Autodesk Fusion 360 part; units mm, degrees
(part 5 of 5)
  arc A59 (-253.4198, 76.6618) -> (-253.4094, 76.4118) centre (-250.4198, 76.6618) ccw
  line L124 (-253.4198, 76.6618) -> (-253.4198, 77.4318)
  arc A60 (-253.4094, 77.6818) -> (-253.4198, 77.4318) centre (-250.4198, 77.4318) ccw
  arc A61 (-253.4198, 77.9318) -> (-253.4094, 77.6818) centre (-250.4198, 77.9318) ccw
  line L125 (-253.4198, 77.9318) -> (-253.4198, 78.7018)
  arc A62 (-253.4094, 78.9518) -> (-253.4198, 78.7018) centre (-250.4198, 78.7018) ccw
  arc A63 (-253.4198, 79.2018) -> (-253.4094, 78.9518) centre (-250.4198, 79.2018) ccw
  line L126 (-253.4198, 79.2018) -> (-253.4198, 79.9718)
  arc A64 (-253.4094, 80.2218) -> (-253.4198, 79.9718) centre (-250.4198, 79.9718) ccw
  arc A65 (-253.4198, 80.4718) -> (-253.4094, 80.2218) centre (-250.4198, 80.4718) ccw
  line L127 (-253.4198, 80.4718) -> (-253.4198, 85.5518)
  arc A66 (-252.4198, 86.5518) -> (-253.4198, 85.5518) centre (-252.4198, 85.5518) ccw
  line L128 (-252.4198, 86.5518) -> (-249.2148, 86.5518)
  arc A67 (-248.9648, 86.5414) -> (-249.2148, 86.5518) centre (-249.2148, 83.5518) ccw
  arc A68 (-248.7148, 86.5518) -> (-248.9648, 86.5414) centre (-248.7148, 83.5518) ccw
  line L129 (-333.4198, 66.966) -> (-333.4198, 73.5518)
  line L130 (-333.4198, 73.5518) -> (-326.834, 73.5518)
  line L131 (-326.834, 73.5518) -> (-333.4198, 66.966)
  line L132 (-323.4198, 72.1376) -> (-316.834, 65.5518)
  line L133 (-316.834, 65.5518) -> (-323.4198, 65.5518)
  line L134 (-323.4198, 65.5518) -> (-323.4198, 72.1376)
  line L135 (-305.4198, 72.1376) -> (-305.4198, 65.5518)
  line L136 (-305.4198, 65.5518) -> (-312.0056, 65.5518)
  line L137 (-312.0056, 65.5518) -> (-305.4198, 72.1376)
  line L138 (-303.4198, 76.966) -> (-303.4198, 83.5518)
  line L139 (-303.4198, 83.5518) -> (-296.834, 83.5518)
  line L140 (-296.834, 83.5518) -> (-303.4198, 76.966)
  line L141 (-285.4198, 65.5518) -> (-292.0056, 65.5518)
  line L142 (-292.0056, 65.5518) -> (-285.4198, 72.1376)
  line L143 (-285.4198, 72.1376) -> (-285.4198, 65.5518)
  line L144 (-283.4198, 83.5518) -> (-276.834, 83.5518)
  line L145 (-276.834, 83.5518) -> (-283.4198, 76.966)
  line L146 (-283.4198, 76.966) -> (-283.4198, 83.5518)
  line L147 (-265.4198, 65.5518) -> (-272.0056, 65.5518)
  line L148 (-272.0056, 65.5518) -> (-265.4198, 72.1376)
  line L149 (-265.4198, 72.1376) -> (-265.4198, 65.5518)
  line L150 (-263.4198, 76.966) -> (-263.4198, 83.5518)
  line L151 (-263.4198, 83.5518) -> (-256.834, 83.5518)
  line L152 (-256.834, 83.5518) -> (-263.4198, 76.966)
  line L153 (-262.0056, 73.5518) -> (-255.4198, 73.5518)
  line L154 (-255.4198, 73.5518) -> (-255.4198, 66.966)
  line L155 (-255.4198, 66.966) -> (-262.0056, 73.5518)
  line L156 (-272.0056, 83.5518) -> (-265.4198, 83.5518)
  line L157 (-265.4198, 83.5518) -> (-265.4198, 76.966)
  line L158 (-265.4198, 76.966) -> (-272.0056, 83.5518)
  line L159 (-282.0056, 73.5518) -> (-275.4198, 73.5518)
  line L160 (-275.4198, 73.5518) -> (-275.4198, 66.966)
  line L161 (-275.4198, 66.966) -> (-282.0056, 73.5518)
  line L162 (-285.4198, 76.966) -> (-292.0056, 83.5518)
  line L163 (-292.0056, 83.5518) -> (-285.4198, 83.5518)
  line L164 (-285.4198, 83.5518) -> (-285.4198, 76.966)
  line L165 (-302.0056, 73.5518) -> (-295.4198, 73.5518)
  line L166 (-295.4198, 73.5518) -> (-295.4198, 66.966)
  line L167 (-295.4198, 66.966) -> (-302.0056, 73.5518)
  line L168 (-305.4198, 76.966) -> (-312.0056, 83.5518)
  line L169 (-312.0056, 83.5518) -> (-305.4198, 83.5518)
  line L170 (-305.4198, 83.5518) -> (-305.4198, 76.966)
  line L171 (-315.4198, 66.966) -> (-322.0056, 73.5518)
  line L172 (-322.0056, 73.5518) -> (-315.4198, 73.5518)
  line L173 (-315.4198, 73.5518) -> (-315.4198, 66.966)
  line L174 (-325.4198, 65.5518) -> (-332.0056, 65.5518)
  line L175 (-332.0056, 65.5518) -> (-325.4198, 72.1376)
  line L176 (-325.4198, 72.1376) -> (-325.4198, 65.5518)
  line L177 (-332.0056, 83.5518) -> (-325.4198, 83.5518)
  line L178 (-325.4198, 83.5518) -> (-325.4198, 76.966)
  line L179 (-325.4198, 76.966) -> (-332.0056, 83.5518)
  line L180 (-323.4198, 76.966) -> (-323.4198, 83.5518)
  line L181 (-323.4198, 83.5518) -> (-316.834, 83.5518)
  line L182 (-316.834, 83.5518) -> (-323.4198, 76.966)
  line L183 (-313.4198, 66.966) -> (-313.4198, 73.5518)
  line L184 (-313.4198, 73.5518) -> (-306.834, 73.5518)
  line L185 (-306.834, 73.5518) -> (-313.4198, 66.966)
  line L186 (-303.4198, 72.1376) -> (-296.834, 65.5518)
  line L187 (-296.834, 65.5518) -> (-303.4198, 65.5518)
  line L188 (-303.4198, 65.5518) -> (-303.4198, 72.1376)
  line L189 (-293.4198, 66.966) -> (-293.4198, 73.5518)
  line L190 (-293.4198, 73.5518) -> (-286.834, 73.5518)
  line L191 (-286.834, 73.5518) -> (-293.4198, 66.966)
  line L192 (-282.0056, 75.5518) -> (-275.4198, 82.1376)
  line L193 (-275.4198, 82.1376) -> (-275.4198, 75.5518)
  line L194 (-275.4198, 75.5518) -> (-282.0056, 75.5518)
  line L195 (-273.4198, 66.966) -> (-273.4198, 73.5518)
  line L196 (-273.4198, 73.5518) -> (-266.834, 73.5518)
  line L197 (-266.834, 73.5518) -> (-273.4198, 66.966)
  line L198 (-262.0056, 75.5518) -> (-255.4198, 82.1376)
  line L199 (-255.4198, 82.1376) -> (-255.4198, 75.5518)
  line L200 (-255.4198, 75.5518) -> (-262.0056, 75.5518)
  line L201 (-263.4198, 65.5518) -> (-263.4198, 72.1376)
  line L202 (-263.4198, 72.1376) -> (-256.834, 65.5518)
  line L203 (-256.834, 65.5518) -> (-263.4198, 65.5518)
  line L204 (-273.4198, 82.1376) -> (-266.834, 75.5518)
  line L205 (-266.834, 75.5518) -> (-273.4198, 75.5518)
  line L206 (-273.4198, 75.5518) -> (-273.4198, 82.1376)
  line L207 (-283.4198, 65.5518) -> (-283.4198, 72.1376)
  line L208 (-283.4198, 72.1376) -> (-276.834, 65.5518)
  line L209 (-276.834, 65.5518) -> (-283.4198, 65.5518)
  line L210 (-293.4198, 82.1376) -> (-286.834, 75.5518)
  line L211 (-286.834, 75.5518) -> (-293.4198, 75.5518)
  line L212 (-293.4198, 75.5518) -> (-293.4198, 82.1376)
  line L213 (-302.0056, 75.5518) -> (-295.4198, 82.1376)
  line L214 (-295.4198, 82.1376) -> (-295.4198, 75.5518)
  line L215 (-295.4198, 75.5518) -> (-302.0056, 75.5518)
  line L216 (-313.4198, 75.5518) -> (-313.4198, 82.1376)
  line L217 (-313.4198, 82.1376) -> (-306.834, 75.5518)
  line L218 (-306.834, 75.5518) -> (-313.4198, 75.5518)
  line L219 (-322.0056, 75.5518) -> (-315.4198, 82.1376)
  line L220 (-315.4198, 82.1376) -> (-315.4198, 75.5518)
  line L221 (-315.4198, 75.5518) -> (-322.0056, 75.5518)
  line L222 (-333.4198, 82.1376) -> (-326.834, 75.5518)
  line L223 (-326.834, 75.5518) -> (-333.4198, 75.5518)
  line L224 (-333.4198, 75.5518) -> (-333.4198, 82.1376)
  line L225 (-278.3217, 111.8636) -> (-280.8652, 114.4071)
  line L226 (-278.3217, 106.2068) -> (-286.4809, 114.3659)
  line L227 (-278.3217, 100.5499) -> (-292.089, 114.3172)
  line L228 (-278.3217, 94.893) -> (-297.693, 114.2643)
  line L229 (-278.3217, 89.2362) -> (-303.3266, 114.2411)
  line L230 (-283.9362, 89.1938) -> (-308.9411, 114.1987)
  line L231 (-289.5507, 89.1515) -> (-314.5556, 114.1564)
  line L232 (-333.4198, 103.3404) -> (-322.6241, 114.1362)
  line L233 (-333.4198, 108.9972) -> (-328.2809, 114.1362)
  line L234 (-325.0115, 89.1213) -> (-311.4909, 102.6419)
  line L235 (-330.6683, 89.1213) -> (-314.3193, 105.4703)
  line L236 (-333.4208, 92.0257) -> (-317.1477, 108.2988)
  line L237 (-333.4198, 97.6835) -> (-319.9762, 111.1272)
  line L238 (-319.3546, 89.1213) -> (-308.6625, 99.8135)
  line L239 (-313.6978, 77.8076) -> (-307.9536, 83.5518)
  line L240 (-302.3841, 89.1213) -> (-300.1772, 91.3282)
  line L241 (-316.5262, 80.636) -> (-315.4198, 81.7424)
  line L242 (-308.0409, 89.1213) -> (-303.0056, 94.1566)
  line L243 (-319.3546, 83.4645) -> (-319.2673, 83.5518)
  line L244 (-313.6978, 89.1213) -> (-305.834, 96.985)
  line L245 (-277.6146, 112.5707) -> (-280.1581, 115.1143)
  line L246 (-279.0288, 111.1565) -> (-281.5724, 113.7)
  line L247 (-277.6146, 106.9139) -> (-285.7738, 115.073)
  line L248 (-279.0288, 105.4996) -> (-287.188, 113.6588)
  line L249 (-277.6146, 101.257) -> (-291.3819, 115.0243)
  line L250 (-279.0288, 99.8428) -> (-292.7961, 113.6101)
  line L251 (-277.6146, 95.6002) -> (-296.9859, 114.9714)
  line L252 (-279.0288, 94.1859) -> (-298.4001, 113.5572)
  line L253 (-277.6146, 89.9433) -> (-302.6195, 114.9482)
  line L254 (-279.0288, 88.5291) -> (-304.0337, 113.534)
  line L255 (-283.2291, 89.9009) -> (-308.234, 114.9058)
  line L256 (-284.6433, 88.4867) -> (-309.6482, 113.4916)
  line L257 (-288.8436, 89.8586) -> (-313.8485, 114.8635)
  line L258 (-290.2578, 88.4444) -> (-315.2627, 113.4493)
  line L259 (-301.677, 88.4142) -> (-299.4701, 90.6211)
  line L260 (-303.0912, 89.8284) -> (-300.8843, 92.0353)
  line L261 (-307.3338, 88.4142) -> (-302.2985, 93.4495)
  line L262 (-308.748, 89.8284) -> (-303.7127, 94.8637)
  line L263 (-312.9907, 88.4142) -> (-305.1269, 96.2779)
  line L264 (-314.4049, 89.8284) -> (-306.5411, 97.6922)
  line L265 (-318.6475, 88.4142) -> (-307.9554, 99.1064)
  line L266 (-320.0617, 89.8284) -> (-309.3696, 100.5206)
  line L267 (-324.3044, 88.4142) -> (-310.7838, 101.9348)
  line L268 (-325.7186, 89.8284) -> (-312.198, 103.349)
  line L269 (-329.9612, 88.4142) -> (-313.6122, 104.7632)
  line L270 (-331.3754, 89.8284) -> (-315.0264, 106.1774)
  line L271 (-332.7137, 91.3186) -> (-316.4406, 107.5916)
  line L272 (-334.1279, 92.7328) -> (-317.8549, 109.0059)
  line L273 (-332.7127, 96.9764) -> (-319.2691, 110.4201)
  line L274 (-334.1269, 98.3906) -> (-320.6833, 111.8343)
  line L275 (-332.7127, 102.6333) -> (-321.917, 113.429)
  line L276 (-334.1269, 104.0475) -> (-323.3312, 114.8433)
  line L277 (-332.7127, 108.2901) -> (-327.5738, 113.429)
  line L278 (-334.1269, 109.7043) -> (-328.988, 114.8433)
  circle A69 centre (-278.3217, 111.8636) radius 1
  circle A70 centre (-280.8652, 114.4071) radius 1
  circle A71 centre (-286.4809, 114.3659) radius 1
  circle A72 centre (-292.089, 114.3172) radius 1
  circle A73 centre (-297.693, 114.2643) radius 1
  circle A74 centre (-303.3266, 114.2411) radius 1
  circle A75 centre (-308.9411, 114.1987) radius 1
  circle A76 centre (-314.5556, 114.1564) radius 1
  circle A77 centre (-328.2809, 114.1362) radius 1
  circle A78 centre (-322.6241, 114.1362) radius 1
  circle A79 centre (-319.9762, 111.1272) radius 1
  circle A80 centre (-317.1477, 108.2988) radius 1
  circle A81 centre (-314.3193, 105.4703) radius 1
  circle A82 centre (-311.4909, 102.6419) radius 1
  circle A83 centre (-308.6625, 99.8135) radius 1
  circle A84 centre (-305.834, 96.985) radius 1
  circle A85 centre (-303.0056, 94.1566) radius 1
  circle A86 centre (-300.1772, 91.3282) radius 1
  circle A87 centre (-333.4198, 97.6835) radius 1
  circle A88 centre (-333.4198, 103.3404) radius 1
  circle A89 centre (-333.4198, 108.9972) radius 1
  circle A90 centre (-333.4208, 92.0257) radius 1
  circle A91 centre (-330.6683, 89.1213) radius 1
  circle A92 centre (-325.0115, 89.1213) radius 1
  circle A93 centre (-319.3546, 89.1213) radius 1
  circle A94 centre (-313.6978, 89.1213) radius 1
  circle A95 centre (-308.0409, 89.1213) radius 1
  circle A96 centre (-302.3841, 89.1213) radius 1
  circle A97 centre (-289.5507, 89.1515) radius 1
  circle A98 centre (-283.9362, 89.1938) radius 1
  circle A99 centre (-278.3217, 89.2362) radius 1
  circle A100 centre (-278.3217, 94.893) radius 1
  circle A101 centre (-278.3217, 100.5499) radius 1
  circle A102 centre (-278.3217, 106.2068) radius 1
  spline S197 degree 3 poles (-269.4518, 103.3713) (-269.4881, 103.3939) (-269.5678, 103.4435) (-269.6619, 103.4471) (-269.713, 103.4491) knots 0 0 0 0 0.012631 0.027679 0.027679 0.027679 0.027679
  spline S198 degree 3 poles (-270.0459, 103.2185) (-270.0428, 103.1922) (-270.0364, 103.1388) (-269.9947, 103.1048) (-269.9736, 103.0875) knots 0 0 0 0 0.007652 0.015492 0.015492 0.015492 0.015492
  spline S199 degree 3 poles (-269.9736, 103.0875) (-269.9445, 103.0745) (-269.8638, 103.0382) (-269.7777, 103.0175) (-269.7226, 103.0043) knots 0 0 0 0 0.009553 0.026493 0.026493 0.026493 0.026493
  spline S200 degree 3 poles (-269.7226, 103.0043) (-269.6457, 102.9851) (-269.5185, 102.9532) (-269.3964, 102.9053) (-269.3481, 102.8863) knots 0 0 0 0 0.023736 0.039299 0.039299 0.039299 0.039299
  spline S201 degree 3 poles (-269.3481, 102.8863) (-269.3157, 102.8686) (-269.2528, 102.8342) (-269.2104, 102.7765) (-269.1898, 102.7485) knots 0 0 0 0 0.010927 0.021211 0.021211 0.021211 0.021211
  spline S202 degree 3 poles (-269.1898, 102.7485) (-269.1741, 102.7183) (-269.1424, 102.6573) (-269.1381, 102.5887) (-269.1359, 102.5541) knots 0 0 0 0 0.010103 0.020373 0.020373 0.020373 0.020373
  spline S203 degree 3 poles (-269.1359, 102.5541) (-269.1377, 102.5225) (-269.1413, 102.46) (-269.1674, 102.403) (-269.1803, 102.3747) knots 0 0 0 0 0.009394 0.018625 0.018625 0.018625 0.018625
  spline S204 degree 3 poles (-269.1803, 102.3747) (-269.1964, 102.3484) (-269.2287, 102.2956) (-269.2769, 102.257) (-269.301, 102.2376) knots 0 0 0 0 0.009191 0.018392 0.018392 0.018392 0.018392
  spline S205 degree 3 poles (-269.301, 102.2376) (-269.3232, 102.2237) (-269.372, 102.1929) (-269.4271, 102.1755) (-269.4572, 102.166) knots 0 0 0 0 0.007816 0.017247 0.017247 0.017247 0.017247
  line L279 (-270.6352, 51.6914) -> (-270.3788, 51.6914)
  spline S206 degree 3 poles (-271.2001, 103.4491) (-271.2429, 103.4465) (-271.3256, 103.4416) (-271.3964, 103.3988) (-271.4306, 103.3781) knots 0 0 0 0 0.012642 0.024448 0.024448 0.024448 0.024448
  spline S207 degree 3 poles (-271.6134, 103.5282) (-271.5534, 103.564) (-271.4259, 103.6399) (-271.2773, 103.6472) (-271.1987, 103.651) knots 0 0 0 0 0.020652 0.043844 0.043844 0.043844 0.043844
  spline S208 degree 3 poles (-270.6967, 102.3386) (-270.7652, 102.2797) (-270.9056, 102.1591) (-271.0905, 102.1442) (-271.1851, 102.1367) knots 0 0 0 0 0.026399 0.05408 0.05408 0.05408 0.05408
  spline S209 degree 3 poles (-271.1851, 102.1367) (-271.2768, 102.1442) (-271.4567, 102.159) (-271.593, 102.2768) (-271.6598, 102.3345) knots 0 0 0 0 0.026858 0.052633 0.052633 0.052633 0.052633
  spline S210 degree 3 poles (-271.6598, 102.3345) (-271.7135, 102.4112) (-271.8298, 102.5776) (-271.839, 102.7813) (-271.844, 102.8911) knots 0 0 0 0 0.027523 0.05971 0.05971 0.05971 0.05971
  spline S211 degree 3 poles (-271.844, 102.8911) (-271.8439, 102.9002) (-271.8437, 102.922) (-271.843, 102.9438) (-271.8426, 102.9566) knots 0 0 0 0 0.002729 0.00655 0.00655 0.00655 0.00655
  line L280 (-271.8426, 102.9566) -> (-270.7621, 102.9566)
  spline S212 degree 3 poles (-270.7621, 102.9566) (-270.7692, 103.0293) (-270.7823, 103.1635) (-270.8611, 103.2724) (-270.8972, 103.3222) knots 0 0 0 0 0.021465 0.039604 0.039604 0.039604 0.039604
  spline S213 degree 3 poles (-272.4886, 103.3904) (-272.5003, 103.3956) (-272.527, 103.4073) (-272.5562, 103.4078) (-272.5725, 103.4081) knots 0 0 0 0 0.003804 0.008651 0.008651 0.008651 0.008651
  spline S214 degree 3 poles (-272.7158, 103.6155) (-272.6831, 103.6219) (-272.6218, 103.6338) (-272.5594, 103.6362) (-272.5302, 103.6373) knots 0 0 0 0 0.009958 0.018706 0.018706 0.018706 0.018706
  spline S215 degree 3 poles (-272.2192, 103.4839) (-272.2105, 103.4484) (-272.1875, 103.3534) (-272.1885, 103.2553) (-272.1892, 103.194) knots 0 0 0 0 0.010927 0.02924 0.02924 0.02924 0.02924
  line L281 (-272.1892, 103.194) -> (-272.1892, 102.3604)
  line L282 (-272.1892, 102.3604) -> (-272.0091, 102.3604)
  line L283 (-272.0091, 102.3604) -> (-272.0091, 102.1694)
  line L284 (-272.0091, 102.1694) -> (-272.1892, 102.1694)
  line L285 (-272.1892, 102.1694) -> (-272.1892, 101.8106)
  line L286 (-272.1892, 101.8106) -> (-272.4334, 101.6633)
  line L287 (-272.4334, 101.6633) -> (-272.4334, 102.1694)
  line L288 (-272.4334, 102.1694) -> (-272.6803, 102.1694)
  line L289 (-272.6803, 102.1694) -> (-272.6803, 102.3604)
  line L290 (-272.6803, 102.3604) -> (-272.4334, 102.3604)
  line L291 (-272.4334, 102.3604) -> (-272.4334, 103.2076)
  spline S216 degree 3 poles (-272.4334, 103.2076) (-272.433, 103.2365) (-272.4324, 103.2821) (-272.4426, 103.3265) (-272.4463, 103.3427) knots 0 0 0 0 0.008635 0.013608 0.013608 0.013608 0.013608
  spline S217 degree 3 poles (-272.4463, 103.3427) (-272.4514, 103.3522) (-272.4616, 103.3715) (-272.4795, 103.384) (-272.4886, 103.3904) knots 0 0 0 0 0.003189 0.00646 0.00646 0.00646 0.00646
  line L292 (-265.9218, 102.7301) -> (-265.9218, 103.6182)
  line L293 (-265.6571, 101.6182) -> (-266.5439, 101.6182)
  spline S218 degree 3 poles (-266.5439, 101.6182) (-266.6229, 101.6188) (-266.7608, 101.6199) (-266.8937, 101.6565) (-266.9504, 101.6721) knots 0 0 0 0 0.023572 0.041164 0.041164 0.041164 0.041164
  spline S219 degree 3 poles (-267.256, 102.1639) (-267.2506, 102.2317) (-267.2401, 102.365) (-267.1584, 102.4707) (-267.1182, 102.5227) knots 0 0 0 0 0.019911 0.039185 0.039185 0.039185 0.039185
  line L294 (-267.0868, 103.6182) -> (-266.8222, 103.2021)
  spline S220 degree 3 poles (-266.8222, 103.2021) (-266.7876, 103.1487) (-266.7268, 103.0548) (-266.66, 102.9652) (-266.6312, 102.9266) knots 0 0 0 0 0.019089 0.033538 0.033538 0.033538 0.033538
  spline S221 degree 3 poles (-266.6312, 102.9266) (-266.6086, 102.8983) (-266.5688, 102.8486) (-266.5185, 102.8097) (-266.4968, 102.7929) knots 0 0 0 0 0.010792 0.019015 0.019015 0.019015 0.019015
  spline S222 degree 3 poles (-266.4968, 102.7929) (-266.4772, 102.7812) (-266.4392, 102.7584) (-266.3967, 102.7458) (-266.3761, 102.7397) knots 0 0 0 0 0.006806 0.01324 0.01324 0.01324 0.01324
  spline S223 degree 3 poles (-266.3761, 102.7397) (-266.3563, 102.7369) (-266.3075, 102.7301) (-266.2581, 102.7301) (-266.2287, 102.7301) knots 0 0 0 0 0.005978 0.01478 0.01478 0.01478 0.01478
  line L295 (-266.2287, 102.7301) -> (-265.9218, 102.7301)
  line L296 (-268.8917, 102.9566) -> (-267.8113, 102.9566)
  spline S224 degree 3 poles (-267.8113, 102.9566) (-267.8184, 103.0293) (-267.8314, 103.1635) (-267.9102, 103.2724) (-267.9463, 103.3222) knots 0 0 0 0 0.021465 0.039604 0.039604 0.039604 0.039604
  line L297 (-270.2437, 102.5432) -> (-270.0036, 102.5759)
  spline S225 degree 3 poles (-269.9088, 102.4013) (-269.878, 102.3831) (-269.81, 102.3427) (-269.7306, 102.34) (-269.6871, 102.3386) knots 0 0 0 0 0.01057 0.023371 0.023371 0.023371 0.023371
  spline S226 degree 3 poles (-269.6871, 102.3386) (-269.6377, 102.339) (-269.5526, 102.3396) (-269.4772, 102.3783) (-269.4456, 102.3945) knots 0 0 0 0 0.014562 0.025087 0.025087 0.025087 0.025087
  spline S227 degree 3 poles (-269.4456, 102.3945) (-269.4246, 102.4131) (-269.3847, 102.4484) (-269.377, 102.5008) (-269.3733, 102.5255) knots 0 0 0 0 0.00814 0.015395 0.015395 0.015395 0.015395
  spline S228 degree 3 poles (-269.3733, 102.5255) (-269.3746, 102.541) (-269.3772, 102.5723) (-269.3946, 102.5983) (-269.4033, 102.6114) knots 0 0 0 0 0.004598 0.009239 0.009239 0.009239 0.009239
  spline S229 degree 3 poles (-269.4033, 102.6114) (-269.4156, 102.6243) (-269.4423, 102.6526) (-269.4781, 102.6684) (-269.4975, 102.6769) knots 0 0 0 0 0.005284 0.01157 0.01157 0.01157 0.01157
  spline S230 degree 3 poles (-269.4975, 102.6769) (-269.5217, 102.6845) (-269.5935, 102.7071) (-269.6662, 102.7267) (-269.7144, 102.7397) knots 0 0 0 0 0.007605 0.022583 0.022583 0.022583 0.022583
  spline S231 degree 3 poles (-269.7144, 102.7397) (-269.7886, 102.7594) (-269.9115, 102.792) (-270.0307, 102.8361) (-270.078, 102.8536) knots 0 0 0 0 0.023005 0.038118 0.038118 0.038118 0.038118
  spline S232 degree 3 poles (-270.078, 102.8536) (-270.1102, 102.8697) (-270.1733, 102.9012) (-270.2179, 102.9558) (-270.2396, 102.9825) knots 0 0 0 0 0.010681 0.020888 0.020888 0.020888 0.020888
  spline S233 degree 3 poles (-270.2396, 102.9825) (-270.2567, 103.0134) (-270.2928, 103.0787) (-270.2964, 103.1533) (-270.2983, 103.1926) knots 0 0 0 0 0.010453 0.022074 0.022074 0.022074 0.022074
  spline S234 degree 3 poles (-270.2983, 103.1926) (-270.2951, 103.2332) (-270.2887, 103.3156) (-270.2476, 103.3874) (-270.2267, 103.4238) knots 0 0 0 0 0.012054 0.024479 0.024479 0.024479 0.024479
  spline S235 degree 3 poles (-270.2267, 103.4238) (-270.1994, 103.4582) (-270.1431, 103.5295) (-270.0619, 103.5704) (-270.02, 103.5916) knots 0 0 0 0 0.013001 0.026908 0.026908 0.026908 0.026908
  spline S236 degree 3 poles (-271.5097, 51.6887) (-271.4771, 51.6951) (-271.4158, 51.707) (-271.3534, 51.7094) (-271.3242, 51.7105) knots 0 0 0 0 0.009958 0.018706 0.018706 0.018706 0.018706
  spline S237 degree 3 poles (-271.3242, 51.7105) (-271.284, 51.7098) (-271.2121, 51.7084) (-271.146, 51.6805) (-271.1168, 51.6682) knots 0 0 0 0 0.011916 0.021334 0.021334 0.021334 0.021334
  spline S238 degree 3 poles (-271.1168, 51.6682) (-271.0943, 51.6534) (-271.0506, 51.6248) (-271.0253, 51.5791) (-271.0131, 51.557) knots 0 0 0 0 0.007958 0.015408 0.015408 0.015408 0.015408
  spline S239 degree 3 poles (-271.0131, 51.557) (-271.0045, 51.5215) (-270.9814, 51.4265) (-270.9825, 51.3285) (-270.9831, 51.2671) knots 0 0 0 0 0.010927 0.02924 0.02924 0.02924 0.02924
  line L298 (-270.9831, 51.2671) -> (-270.9831, 50.4336)
  line L299 (-270.9831, 50.4336) -> (-270.803, 50.4336)
  line L300 (-270.803, 50.4336) -> (-270.803, 50.2426)
  line L301 (-270.803, 50.2426) -> (-270.9831, 50.2426)
  line L302 (-270.9831, 50.2426) -> (-270.9831, 49.8838)
  line L303 (-270.9831, 49.8838) -> (-271.2273, 49.7364)
  line L304 (-271.2273, 49.7364) -> (-271.2273, 50.2426)
  line L305 (-271.2273, 50.2426) -> (-271.4743, 50.2426)
  line L306 (-271.4743, 50.2426) -> (-271.4743, 50.4336)
  line L307 (-271.4743, 50.4336) -> (-271.2273, 50.4336)
  line L308 (-271.2273, 50.4336) -> (-271.2273, 51.2808)
  spline S240 degree 3 poles (-271.2273, 51.2808) (-271.227, 51.3097) (-271.2264, 51.3553) (-271.2366, 51.3996) (-271.2403, 51.4158) knots 0 0 0 0 0.008635 0.013608 0.013608 0.013608 0.013608
  spline S241 degree 3 poles (-271.2403, 51.4158) (-271.2454, 51.4254) (-271.2556, 51.4447) (-271.2735, 51.4572) (-271.2826, 51.4636) knots 0 0 0 0 0.003189 0.00646 0.00646 0.00646 0.00646
  spline S242 degree 3 poles (-269.301, 51.3094) (-269.3029, 51.275) (-269.3066, 51.207) (-269.3353, 51.1454) (-269.3494, 51.115) knots 0 0 0 0 0.010253 0.020199 0.020199 0.020199 0.020199
  spline S243 degree 3 poles (-269.3494, 51.115) (-269.3666, 51.0873) (-269.4005, 51.0326) (-269.4513, 50.9932) (-269.4763, 50.9738) knots 0 0 0 0 0.009704 0.019119 0.019119 0.019119 0.019119
  spline S244 degree 3 poles (-269.4763, 50.9738) (-269.5036, 50.9571) (-269.5591, 50.923) (-269.6213, 50.9033) (-269.653, 50.8933) knots 0 0 0 0 0.009559 0.019479 0.019479 0.019479 0.019479
  spline S245 degree 3 poles (-269.653, 50.8933) (-269.6832, 50.8867) (-269.7553, 50.8708) (-269.8286, 50.8617) (-269.8713, 50.8565) knots 0 0 0 0 0.009264 0.022147 0.022147 0.022147 0.022147
  spline S246 degree 3 poles (-269.8713, 50.8565) (-269.9578, 50.846) (-270.1059, 50.8281) (-270.2495, 50.7884) (-270.3092, 50.7719) knots 0 0 0 0 0.02611 0.044656 0.044656 0.044656 0.044656
  spline S247 degree 3 poles (-270.3092, 50.7719) (-270.3096, 50.7582) (-270.3102, 50.7368) (-270.3105, 50.7154) (-270.3106, 50.7078) knots 0 0 0 0 0.004128 0.006414 0.006414 0.006414 0.006414
  spline S248 degree 3 poles (-270.3106, 50.7078) (-270.3096, 50.6634) (-270.3078, 50.5852) (-270.2612, 50.5232) (-270.241, 50.4963) knots 0 0 0 0 0.012908 0.022759 0.022759 0.022759 0.022759
  spline S249 degree 3 poles (-270.241, 50.4963) (-270.2031, 50.4721) (-270.1183, 50.418) (-270.0172, 50.4149) (-269.9613, 50.4131) knots 0 0 0 0 0.013259 0.029661 0.029661 0.029661 0.029661
  spline S250 degree 3 poles (-269.9613, 50.4131) (-269.91, 50.4139) (-269.8198, 50.4153) (-269.7399, 50.4562) (-269.7055, 50.4738) knots 0 0 0 0 0.015134 0.026599 0.026599 0.026599 0.026599
  spline S251 degree 3 poles (-269.7055, 50.4738) (-269.6792, 50.5004) (-269.6196, 50.5608) (-269.5964, 50.6428) (-269.5834, 50.6887) knots 0 0 0 0 0.011056 0.025069 0.025069 0.025069 0.025069
  line L309 (-269.5834, 50.6887) -> (-269.3433, 50.656)
  spline S252 degree 3 poles (-269.3433, 50.656) (-269.355, 50.6083) (-269.3769, 50.5191) (-269.4275, 50.4426) (-269.4511, 50.407) knots 0 0 0 0 0.01459 0.02731 0.02731 0.02731 0.02731
  spline S253 degree 3 poles (-269.4511, 50.407) (-269.4801, 50.3768) (-269.5418, 50.3126) (-269.6243, 50.2789) (-269.668, 50.261) knots 0 0 0 0 0.012433 0.026404 0.026404 0.026404 0.026404
  spline S254 degree 3 poles (-270.5732, 51.5175) (-270.5797, 51.5475) (-270.593, 51.6082) (-270.6211, 51.6635) (-270.6352, 51.6914) knots 0 0 0 0 0.009187 0.018535 0.018535 0.018535 0.018535
  spline S255 degree 3 poles (-271.1987, 103.651) (-271.0998, 103.6444) (-270.9107, 103.6319) (-270.7644, 103.5123) (-270.6946, 103.4552) knots 0 0 0 0 0.028913 0.055291 0.055291 0.055291 0.055291
  spline S256 degree 3 poles (-270.6946, 103.4552) (-270.6404, 103.3795) (-270.5232, 103.2161) (-270.5136, 103.0144) (-270.5084, 102.9061) knots 0 0 0 0 0.027351 0.059089 0.059089 0.059089 0.059089
  spline S257 degree 3 poles (-270.5084, 102.9061) (-270.5135, 102.7942) (-270.523, 102.5864) (-270.6418, 102.4168) (-270.6967, 102.3386) knots 0 0 0 0 0.032809 0.060899 0.060899 0.060899 0.060899
  spline S258 degree 3 poles (-270.8972, 103.3222) (-270.9405, 103.3592) (-271.0278, 103.4339) (-271.1423, 103.444) (-271.2001, 103.4491) knots 0 0 0 0 0.016633 0.033577 0.033577 0.033577 0.033577
  spline S259 degree 3 poles (-272.5302, 103.6373) (-272.4901, 103.6366) (-272.4181, 103.6352) (-272.352, 103.6073) (-272.3229, 103.595) knots 0 0 0 0 0.011916 0.021334 0.021334 0.021334 0.021334
  spline S260 degree 3 poles (-272.3229, 103.595) (-272.3003, 103.5802) (-272.2566, 103.5516) (-272.2314, 103.5059) (-272.2192, 103.4839) knots 0 0 0 0 0.007958 0.015408 0.015408 0.015408 0.015408
  spline S261 degree 3 poles (-267.1182, 102.5227) (-267.062, 102.5674) (-266.9372, 102.6667) (-266.7793, 102.6935) (-266.6926, 102.7083) knots 0 0 0 0 0.021209 0.047103 0.047103 0.047103 0.047103
  spline S262 degree 3 poles (-266.6926, 102.7083) (-266.7241, 102.7239) (-266.7806, 102.7518) (-266.8302, 102.7907) (-266.8522, 102.8079) knots 0 0 0 0 0.010515 0.018858 0.018858 0.018858 0.018858
  spline S263 degree 3 poles (-266.8522, 102.8079) (-266.8911, 102.8467) (-266.9728, 102.9283) (-267.0378, 103.0239) (-267.0718, 103.0739) knots 0 0 0 0 0.016455 0.034567 0.034567 0.034567 0.034567
  line L310 (-267.0718, 103.0739) -> (-267.4197, 103.6182)
  line L311 (-267.4197, 103.6182) -> (-267.0868, 103.6182)
  dimension "d167" = 1
  dimension "d168" = -1
  dimension "d169" = 1
  dimension "d170" = -1
  dimension "d171" = 1
  dimension "d172" = -1
  dimension "d173" = 1
  dimension "d174" = -1
  dimension "d175" = 1
  dimension "d176" = -1
  dimension "d177" = 1
  dimension "d178" = -1
  dimension "d179" = 1
  dimension "d180" = -1
  dimension "d183" = 1
  dimension "d184" = -1
  dimension "d185" = 1
  dimension "d186" = -1
  dimension "d187" = 1
  dimension "d188" = -1
  dimension "d189" = 1
  dimension "d190" = -1
  dimension "d191" = 1
  dimension "d192" = -1
  dimension "d193" = 1
  dimension "d194" = -1
  dimension "d195" = 1
  dimension "d196" = -1
  dimension "d197" = 1
  dimension "d198" = -1
  dimension "d199" = 1
  dimension "d200" = -1
  dimension "d201" = 1
  dimension "d202" = -1
  constraint coincident L169 L239.end
  constraint collinear L239 L240
  constraint coincident L220 L241.end
  constraint collinear L241 L242
  constraint coincident L181 L243.end
  constraint collinear L243 L244
  constraint coincident L225.start A69.centre
  constraint coincident L246.start A69
  constraint tangent L246 A69
  constraint coincident L225.end A70.centre
  constraint coincident L246.end A70
  constraint tangent L246 A70
  constraint coincident L226.end A71.centre
  constraint coincident L248.end A71
  constraint tangent L248 A71
  constraint coincident L227.end A72.centre
  constraint coincident L250.end A72
  constraint tangent L250 A72
  constraint coincident L228.end A73.centre
  constraint coincident L252.end A73
  constraint tangent L252 A73
  constraint coincident L229.end A74.centre
  constraint coincident L254.end A74
  constraint tangent L254 A74
  constraint coincident L230.end A75.centre
  constraint coincident L256.end A75
  constraint coincident L231.end A76.centre
  constraint coincident L258.end A76
  constraint tangent L258 A76
  constraint coincident L233.end A77.centre
  constraint coincident L278.end A77
  constraint tangent L278 A77
  constraint coincident L232.end A78.centre
  constraint coincident L276.end A78
  constraint coincident L237.end A79.centre
  constraint coincident L274.end A79
  constraint tangent L274 A79
  constraint coincident L236.end A80.centre
  constraint coincident L272.end A80
  constraint tangent L272 A80
  constraint coincident L235.end A81.centre
  constraint coincident L270.end A81
  constraint tangent L270 A81
  constraint coincident L234.end A82.centre
  constraint coincident L268.end A82
  constraint tangent L268 A82
  constraint coincident L238.end A83.centre
  constraint coincident L266.end A83
  constraint tangent L266 A83
  constraint coincident L244.end A84.centre
  constraint coincident L264.end A84
  constraint tangent L264 A84
  constraint coincident L242.end A85.centre
  constraint coincident L262.end A85
  constraint tangent L262 A85
  constraint coincident L240.end A86.centre
  constraint coincident L260.end A86
  constraint tangent L260 A86
  constraint coincident L237.start A87.centre
  constraint coincident L274.start A87
  constraint tangent L274 A87
  constraint coincident L232.start A88.centre
  constraint coincident L276.start A88
  constraint tangent L276 A88
  constraint coincident L233.start A89.centre
  constraint coincident L278.start A89
  constraint tangent L278 A89
  constraint coincident L236.start A90.centre
  constraint coincident L272.start A90
  constraint tangent L272 A90
  constraint coincident L235.start A91.centre
  constraint coincident L270.start A91
  constraint tangent L270 A91
  constraint coincident L234.start A92.centre
  constraint coincident L268.start A92
  constraint tangent L268 A92
  constraint coincident L238.start A93.centre
  constraint coincident L266.start A93
  constraint tangent L266 A93
  constraint coincident L244.start A94.centre
  constraint coincident L264.start A94
  constraint tangent L264 A94
  constraint coincident L242.start A95.centre
  constraint coincident L262.start A95
  constraint tangent L262 A95
  constraint coincident L240.start A96.centre
  constraint coincident L260.start A96
  constraint tangent L260 A96
  constraint coincident L231.start A97.centre
  constraint coincident L258.start A97
  constraint tangent L258 A97
  constraint coincident L230.start A98.centre
  constraint coincident L256.start A98
  constraint tangent L256 A98
  constraint coincident L229.start A99.centre
  constraint coincident L254.start A99
  constraint tangent L254 A99
  constraint coincident L228.start A100.centre
  constraint coincident L252.start A100
  constraint tangent L252 A100
  constraint coincident L227.start A101.centre
  constraint coincident L250.start A101
  constraint tangent L250 A101
  constraint coincident L226.start A102.centre
  constraint coincident L248.start A102
  constraint tangent L248 A102
extrude "Extrude4" cut sketch "Sketch4" against normal blind 2 contours L225 L246 A69 A70 | L225 L245 A69 A70 | A69 | A70 | L226 L248 A71 A102 | L226 L247 A71 A102 | A102 | A71 | L227 L250 A72 A101 | L227 L249 A72 A101 | A101 | A72 | L228 L252 A73 A100 | L228 L251 A73 A100 | A100 | A73 | L229 L254 A74 A99 | L229 L253 A74 A99 | A99 | A74 | L230 L256 A75 A98 | L230 L255 A75 A98 | A98 | A75 | L231 L258 A76 A97 | L231 L257 A76 A97 | A97 | A76 | L232 L276 A78 A88 | L232 L275 A78 A88 | A88 | A78 | L233 L278 A77 A89 | L233 L277 A77 A89 | A89 | A77 | L234 L268 A82 A92 | L234 L267 A82 A92 | A92 | A82 | L235 L270 A81 A91 | L235 L269 A81 A91 | A91 | A81 | L236 L272 A80 A90 | L236 L271 A80 A90 | A90 | A80 | L237 L274 A79 A87 | L237 L273 A79 A87 | A87 | A79 | L238 L266 A83 A93 | L238 L265 A83 A93 | A93 | A83 | L240 L260 A86 A96 | L240 L259 A86 A96 | A96 | A86 | L242 L262 A85 A95 | L242 L261 A85 A95 | A95 | A85 | L244 L264 A84 A94 | L244 L263 A84 A94 | A94 | A84
equation "d92 = 'Status'"
equation "d94 = 'Status'"
equation "d96 = 'Power'"
equation "d98 = 'Boot'"
equation "d100 = 'Reset'"
equation "d168 = -d167"
equation "d170 = -d169"
equation "d172 = -d171"
equation "d174 = -d173"
equation "d176 = -d175"
equation "d178 = -d177"
equation "d180 = -d179"
equation "d184 = -d183"
equation "d186 = -d185"
equation "d188 = -d187"
equation "d190 = -d189"
equation "d192 = -d191"
equation "d194 = -d193"
equation "d196 = -d195"
equation "d198 = -d197"
equation "d200 = -d199"
equation "d202 = -d201"
